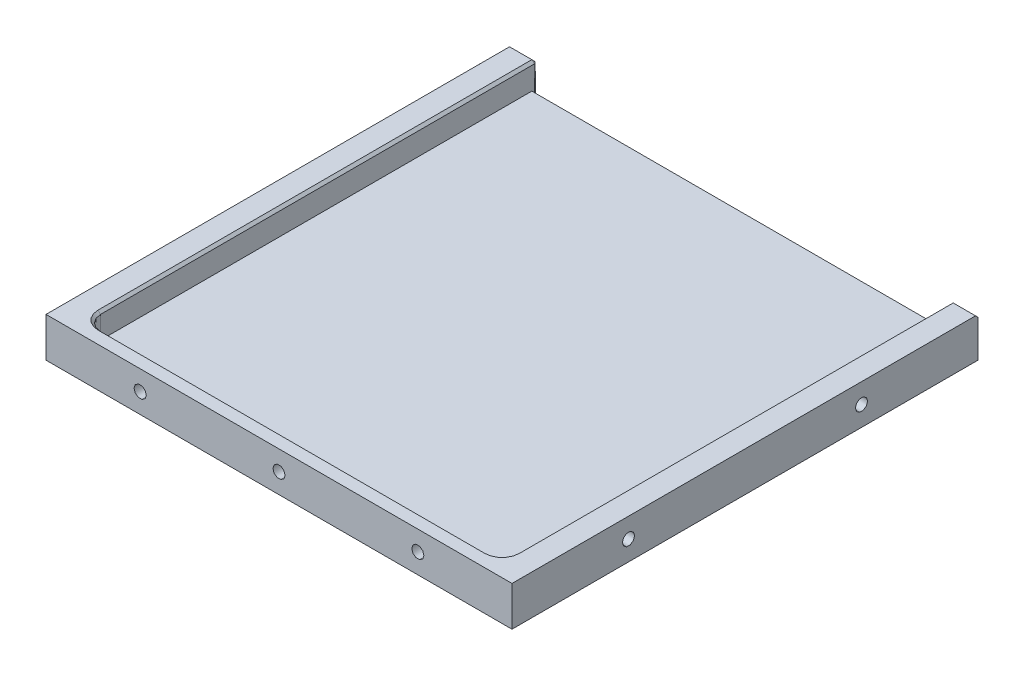
# Autodesk Inventor part: LeftPanel
Saved by Autodesk Inventor 2023 (Build 270158000, 158)
## iProperties
Created: 2022-08-01
Part Number: LeftPanel
Material: Aluminum 6061
Document SubType Name: Modeling
Designer: Aditya Bansal
Density: 2.7 g/cm^3
Appearance: Aluminum - Flat
Mass: 86.8416 g
Surface Area: 217.992 cm^2
Volume: 32.1635 cm^3
Author: Aditya Bansal
Autodesk Inventor part; units mm, degrees
ref_plane "YZ Plane" through (0, 0, 0) normal (1, 0, 0) x (0, 1, 0)
ref_plane "XZ Plane" through (0, 0, 0) normal (0, 1, 0) x (-1, 0, 0)
sketch "Sketch3" plane through (0, 0, 0) normal (0, 1, 0) x (-1, 0, 0)
  line L0 (3, 3) -> (-97, 3) construction
  line L1 (-97, 3) -> (-97, 0) construction
  line L2 (-97, 0) -> (3, 0) construction
  line L3 (3, 0) -> (3, 3) construction
  line L4 (-97, 0) -> (-94, 0) construction
  line L5 (-94, 0) -> (-94, -94) construction
  line L6 (-94, -94) -> (-97, -94) construction
  line L7 (-97, -94) -> (-97, 0) construction
  line L8 (-97, -94) -> (3, -94) construction
  line L9 (3, -94) -> (3, -97) construction
  line L10 (3, -97) -> (-97, -97) construction
  line L11 (-97, -97) -> (-97, -94) construction
  line L12 (3, -94) -> (0, -94) construction
  line L13 (0, -94) -> (0, 0) construction
  line L14 (0, 0) -> (3, 0) construction
  line L15 (3, 0) -> (3, -94) construction
  line L16 (0, -94) -> (-94, -94)
  line L17 (-94, -94) -> (-94, 0)
  line L18 (-94, 0) -> (0, 0)
  line L19 (0, 0) -> (0, -94)
  line L20 (3, 3) -> (3, 0) construction
  dimension "d6" = 3
  dimension "d7" = 100
  dimension "d8" = 100
  dimension "d9" = 3
  constraints: 42 end point, 10 parallel, 5 horizontal, 5 perpendicular, 3 collinear, 2 point on line, 1 coincident, 1 vertical
  measures "d6" distance between parallel lines of L15 L13
  measures "d7" distance between parallel lines of L15 L7
  measures "d8" distance between parallel lines of L10 L0
  measures "d9" distance of L10.end L6.end
extrude "Extrusion2" add sketch "Sketch3" along normal blind 3
sketch "Sketch4" plane through (0, 3, 0) normal (0, 1, 0) x (1, 0, 0)
  line L0 (94, 94) -> (0, 94) projected
  line L1 (0, 0) -> (94, 0) projected
  line L2 (0, 94) -> (5, 94)
  line L3 (5, 94) -> (5, 0)
  line L4 (5, 0) -> (0, 0)
  line L5 (0, 0) -> (0, 94)
  line L6 (94, 0) -> (94, 94) projected
  line L7 (94, 94) -> (89, 94)
  line L8 (89, 94) -> (89, 0)
  line L9 (89, 0) -> (94, 0)
  line L10 (94, 0) -> (94, 94)
  line L11 (5, 3) -> (89, 3)
  line L12 (89, 3) -> (89, 0)
  line L13 (89, 0) -> (5, 0)
  line L14 (5, 0) -> (5, 3)
  dimension "d12" = 5
  dimension "d13" = 3
  constraints: 24 end point, 6 parallel, 4 point on line, 3 horizontal, 3 perpendicular, 1 collinear
  measures "d12" distance between parallel lines of L6 L8
  measures "d13" distance between parallel lines of L1 L11
extrude "Extrusion3" add sketch "Sketch4" along normal blind 5 contours L6 L1 L8 L0 | L3 L1 L5 L0 | L8 L1 L3 L11
sketch "Sketch6" plane through (94, 0, -94) normal (0, 0, -1) x (-1, 0, 0)
  line L0 (0, 0) -> (94, 0) projected
  line L1 (89, 8) -> (94, 8) projected
  line L2 (89, 3) -> (89, 8) projected
  line L3 (94, 0) -> (94, 8) projected
  line L4 (0, 0) -> (0, 8) projected
  point P0 (91.5, 4)
  point P1 (2.5, 4)
  dimension "d28" = 8
  dimension "d29" = 5
  dimension "d30" = 2.5
  dimension "d31" = 4
  dimension "d32" = 2.5
  constraints: 1 horizontal alignment
  measures "d28" distance between parallel lines of L0 L1
  measures "d29" distance between parallel lines of L2 L3
  measures "d30" distance from line of point (91.5, 4) L3
  measures "d31" distance from line of L0 point (91.5, 4)
  measures "d32" distance from line of L4 point (2.5, 4)
hole "Hole1" at (2.5, 4, -94) at (91.5, 4, -94) direction (0, 0, 1) diameter 2.6416 depth 10.979 tip angle 118 thread size "6-32 UNC" class "2B" standard "ANSI Unified Screw Threads"
fillet "Fillet1" radius 3 2 edges at (89, 5.5, -3) (5, 5.5, -3)
fillet "Fillet2" radius 0.5 2 edges at (5, 5.5, -94) (89, 5.5, -94)
sketch "Sketch7" plane through (0, 0, 0) normal (0, 0, 1) x (1, 0, 0)
  line L0 (0, 0) -> (94, 0) projected
  line L1 (0, 0) -> (0, 8) projected
  line L2 (89, 8) -> (5, 8) projected
  point P0 (19, 4)
  point P1 (47, 4)
  point P2 (75, 4)
  dimension "d40" = 4
  dimension "d57" = 84
  dimension "d58" = 14
  dimension "d59" = 28
  dimension "d60" = 28
  constraints: 2 horizontal alignment
  measures "d40" distance from line of point (19, 4) L0
  measures "d57" distance of L2.start L2.end
  measures "d58" horizontal distance of point (19, 4) L2.end
  measures "d59" distance of point (47, 4) point (19, 4)
  measures "d60" distance of point (75, 4) point (47, 4)
hole "Hole2" at (19, 4, 0) at (47, 4, 0) at (75, 4, 0) direction (0, 0, -1) diameter 2.459 depth 3.5 tip angle 118 thread size "M3x0.5" class "6H" standard "ANSI Metric M Profile"
sketch "Sketch9" plane through (0, 0, -94) normal (-1, 0, 0) x (0, 0, 1)
  line L0 (0, 8) -> (94, 8) projected
  line L1 (0, 0) -> (94, 0) projected
  line L2 (0, 0) -> (0, 8) projected
  point P0 (23.5, 4)
  point P1 (70.5, 4)
  dimension "d51" = 4
  dimension "d52" = 8
  dimension "d53" = 94
  dimension "d54" = 23.5
  dimension "d55" = 47
  constraints: 1 horizontal alignment
  measures "d51" distance from line of L0 point (23.5, 4)
  measures "d52" distance between parallel lines of L0 L1
  measures "d53" distance of L0.start L0.end
  measures "d54" distance from line of point (23.5, 4) L2
  measures "d55" distance of point (70.5, 4) point (23.5, 4)
hole "Hole3" at (0, 4, -70.5) at (0, 4, -23.5) direction (1, 0, 0) diameter 2.459 depth 4 tip angle 118 thread size "M3x0.5" class "6H" standard "ANSI Metric M Profile"
ref_plane "Work Plane1" through (47, 0, -94) normal (-1, 0, 0) x (0, 0, 1)
mirror "Mirror1" about plane through (47, 0, -94) normal (-1, 0, 0) of "Hole3"
chamfer "Chamfer2" distance 1 angle 45 1 edges at (47, 3, -94)
chamfer "Chamfer3" distance 0.5 angle 45 3 edges at (5, 8, -49.75) (47, 8, -3) (89, 8, -49.75)
ref_plane "Work Plane2" through (47, 0, -94) normal (-1, 0, 0) x (0, 0, 1)
equation "\"d30\" = 0.5 * d29"
equation "\"d31\" = 0.5 * d28"
equation "\"d32\" = d30"
equation "\"d58\" = 0.166667 * d57"
equation "\"d59\" = 2 * d58"
equation "\"d60\" = d59"
equation "\"d51\" = 0.5 * d52"
equation "\"d54\" = 0.25 * d53"
equation "\"d55\" = 2 * d54"
body "Solid2"
